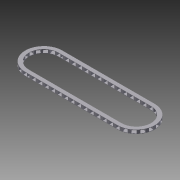
# Autodesk Inventor part: chain
Saved by Autodesk Inventor 2011 (Build 150239000, 239)
## iProperties
Created: 2010-04-19
Part Number: chain
Document SubType Name: Modeling
Designer: lucio
Density: 2.71 g/cm^3
Material: Aluminum-6061
Mass: 13.7583 g
Surface Area: 102.226 cm^2
Volume: 5.07686 cm^3
Author: lucio
Autodesk Inventor part; units mm, degrees
ref_plane "YZ Plane" through (0, 0, 0) normal (1, 0, 0) x (0, 1, 0)
ref_plane "XZ Plane" through (0, 0, 0) normal (0, 1, 0) x (-1, 0, 0)
ref_plane "XY Plane" through (0, 0, 0) normal (0, 0, 1) x (1, 0, 0)
sketch "Sketch1" plane through (0, 0, 0) normal (0, 0, 1) x (1, 0, 0)
  line L0 (25, 0) -> (150, 0)
  line L1 (175, 25) -> (175, 25)
  line L2 (150, 50) -> (25, 50)
  line L3 (0, 25) -> (0, 25)
  arc A0 (25, 50) -> (0, 25) centre (25, 25) ccw
  arc A1 (175, 25) -> (150, 50) centre (150, 25) ccw
  arc A2 (150, 0) -> (175, 25) centre (150, 25) ccw
  arc A3 (0, 25) -> (25, 0) centre (25, 25) ccw
  line L4 (25, 45) -> (150, 45)
  line L5 (170, 25) -> (170, 25)
  line L6 (150, 5) -> (25, 5)
  line L7 (5, 25) -> (5, 25)
  arc A4 (25, 45) -> (5, 25) centre (25, 25) ccw
  arc A5 (5, 25) -> (25, 5) centre (25, 25) ccw
  arc A6 (150, 5) -> (170, 25) centre (150, 25) ccw
  arc A7 (170, 25) -> (150, 45) centre (150, 25) ccw
  line L8 (22.5, 25) -> (27.5, 25)
  line L9 (27.5, 25) -> (27.5, 50)
  line L10 (27.5, 50) -> (22.5, 50)
  line L11 (22.5, 50) -> (22.5, 25)
  line L12 (22.650768, 24.14495) -> (27.349232, 25.85505)
  line L13 (27.349232, 25.85505) -> (18.798728, 49.347366)
  line L14 (18.798728, 49.347366) -> (14.100265, 47.637265)
  line L15 (14.100265, 47.637265) -> (22.650768, 24.14495)
  line L16 (23.084889, 23.393031) -> (26.915111, 26.606969)
  line L17 (26.915111, 26.606969) -> (10.845421, 45.75808)
  line L18 (10.845421, 45.75808) -> (7.015199, 42.544142)
  line L19 (7.015199, 42.544142) -> (23.084889, 23.393031)
  line L20 (23.75, 22.834936) -> (26.25, 27.165064)
  line L21 (26.25, 27.165064) -> (4.599365, 39.665064)
  line L22 (4.599365, 39.665064) -> (2.099365, 35.334936)
  line L23 (2.099365, 35.334936) -> (23.75, 22.834936)
  line L24 (24.56588, 22.537981) -> (25.43412, 27.462019)
  line L25 (25.43412, 27.462019) -> (0.813927, 31.803224)
  line L26 (0.813927, 31.803224) -> (-0.054314, 26.879185)
  line L27 (-0.054314, 26.879185) -> (24.56588, 22.537981)
  line L28 (25.43412, 22.537981) -> (24.56588, 27.462019)
  line L29 (24.56588, 27.462019) -> (-0.054314, 23.120815)
  line L30 (-0.054314, 23.120815) -> (0.813927, 18.196776)
  line L31 (0.813927, 18.196776) -> (25.43412, 22.537981)
  line L32 (26.25, 22.834936) -> (23.75, 27.165064)
  line L33 (23.75, 27.165064) -> (2.099365, 14.665064)
  line L34 (2.099365, 14.665064) -> (4.599365, 10.334936)
  line L35 (4.599365, 10.334936) -> (26.25, 22.834936)
  line L36 (26.915111, 23.393031) -> (23.084889, 26.606969)
  line L37 (23.084889, 26.606969) -> (7.015199, 7.455858)
  line L38 (7.015199, 7.455858) -> (10.845421, 4.24192)
  line L39 (10.845421, 4.24192) -> (26.915111, 23.393031)
  line L40 (27.349232, 24.14495) -> (22.650768, 25.85505)
  line L41 (22.650768, 25.85505) -> (14.100265, 2.362735)
  line L42 (14.100265, 2.362735) -> (18.798728, 0.652634)
  line L43 (18.798728, 0.652634) -> (27.349232, 24.14495)
  line L44 (27.5, 25) -> (22.5, 25)
  line L45 (22.5, 25) -> (22.5, 0)
  line L46 (22.5, 0) -> (27.5, 0)
  line L47 (27.5, 0) -> (27.5, 25)
  line L48 (147.5, 24.96674) -> (152.5, 24.96674)
  line L49 (152.5, 24.96674) -> (152.5, 51.038636)
  line L50 (152.082241, 51.032629) -> (147.5, 50.96674)
  line L51 (147.5, 50.96674) -> (147.5, 24.96674)
  line L52 (147.639393, 25.823796) -> (152.337856, 24.113695)
  line L53 (152.337856, 24.113695) -> (161.254969, 48.613263)
  line L54 (161.254969, 48.613263) -> (156.531917, 50.255804)
  line L55 (156.531917, 50.255804) -> (147.639393, 25.823796)
  line L56 (148.06351, 26.58149) -> (151.893732, 23.367552)
  line L57 (151.893732, 23.367552) -> (168.652423, 43.339783)
  line L58 (168.652423, 43.339783) -> (164.775988, 46.498646)
  line L59 (164.775988, 46.498646) -> (148.06351, 26.58149)
  line L60 (148.721196, 27.148433) -> (151.221196, 22.818306)
  line L61 (151.221196, 22.818306) -> (173.80012, 35.854254)
  line L62 (173.80012, 35.854254) -> (171.237856, 40.148433)
  line L63 (171.237856, 40.148433) -> (148.721196, 27.148433)
  line L64 (149.533125, 27.456244) -> (150.401366, 22.532205)
  line L65 (150.401366, 22.532205) -> (176.077171, 27.059542)
  line L66 (176.077171, 27.059542) -> (175.138126, 31.971096)
  line L67 (175.138126, 31.971096) -> (149.533125, 27.456244)
  line L68 (150.401366, 27.467795) -> (149.533125, 22.543756)
  line L69 (149.533125, 22.543756) -> (175.20893, 18.016419)
  line L70 (175.20893, 18.016419) -> (176.006367, 22.952942)
  line L71 (176.006367, 22.952942) -> (150.401366, 27.467795)
  line L72 (151.221196, 27.181694) -> (148.721196, 22.851567)
  line L73 (148.721196, 22.851567) -> (171.30012, 9.815619)
  line L74 (171.30012, 9.815619) -> (173.737856, 14.181694)
  line L75 (173.737856, 14.181694) -> (151.221196, 27.181694)
  line L76 (151.893732, 26.632448) -> (148.06351, 23.41851)
  line L77 (148.06351, 23.41851) -> (164.822201, 3.446279)
  line L78 (164.822201, 3.446279) -> (168.60621, 6.715292)
  line L79 (168.60621, 6.715292) -> (151.893732, 26.632448)
  line L80 (152.337856, 25.886305) -> (147.639393, 24.176204)
  line L81 (147.639393, 24.176204) -> (156.556506, -0.323364)
  line L82 (156.556506, -0.323364) -> (161.23038, 1.454297)
  line L83 (161.23038, 1.454297) -> (152.337856, 25.886305)
  line L84 (152.5, 25.03326) -> (147.5, 25.03326)
  line L85 (147.5, 25.03326) -> (147.5, -1.038636)
  line L86 (147.5, -1.038636) -> (152.5, -0.96674)
  line L87 (152.5, -0.96674) -> (152.5, 25.03326)
  line L88 (143.785, 50) -> (138.785, 50)
  line L89 (138.785, 50) -> (138.785, -0.715226)
  line L90 (138.785, -0.715226) -> (143.785, -0.715226)
  line L91 (143.785, -0.715226) -> (143.785, 50)
  line L92 (135.07, 50) -> (130.07, 50)
  line L93 (130.07, 50) -> (130.07, 0)
  line L94 (130.07, 0) -> (135.07, 0)
  line L95 (135.07, 0) -> (135.07, 50)
  line L96 (126.355, 0) -> (121.355, 0)
  line L97 (121.355, 0) -> (121.355, 50)
  line L98 (121.355, 50) -> (126.355, 50)
  line L99 (126.355, 50) -> (126.355, 0)
  line L100 (117.64, 50) -> (112.64, 50)
  line L101 (112.64, 50) -> (112.64, 0)
  line L102 (112.64, 0) -> (117.64, 0)
  line L103 (117.64, 0) -> (117.64, 50)
  line L104 (108.925, 50) -> (103.925, 50)
  line L105 (103.925, 50) -> (103.925, 0)
  line L106 (103.925, 0) -> (108.925, 0)
  line L107 (108.925, 0) -> (108.925, 50)
  line L108 (100.21, 50) -> (95.21, 50)
  line L109 (95.21, 50) -> (95.21, 0)
  line L110 (95.21, 0) -> (100.21, 0)
  line L111 (100.21, 0) -> (100.21, 50)
  line L112 (91.495, 50) -> (86.495, 50)
  line L113 (86.495, 50) -> (86.495, 0)
  line L114 (86.495, 0) -> (91.495, 0)
  line L115 (91.495, 0) -> (91.495, 50)
  line L116 (82.78, 50) -> (77.78, 50)
  line L117 (77.78, 50) -> (77.78, 0)
  line L118 (77.78, 0) -> (82.78, 0)
  line L119 (82.78, 0) -> (82.78, 50)
  line L120 (74.065, 50) -> (69.065, 50)
  line L121 (69.065, 50) -> (69.065, 0)
  line L122 (69.065, 0) -> (74.065, 0)
  line L123 (74.065, 0) -> (74.065, 50)
  line L124 (65.35, 50) -> (60.35, 50)
  line L125 (60.35, 50) -> (60.35, 0)
  line L126 (60.35, 0) -> (65.35, 0)
  line L127 (65.35, 0) -> (65.35, 50)
  line L128 (56.635, 50) -> (51.635, 50)
  line L129 (51.635, 50) -> (51.635, 0)
  line L130 (51.635, 0) -> (56.635, 0)
  line L131 (56.635, 0) -> (56.635, 50)
  line L132 (47.92, 50) -> (42.92, 50)
  line L133 (42.92, 50) -> (42.92, 0)
  line L134 (42.92, 0) -> (47.92, 0)
  line L135 (47.92, 0) -> (47.92, 50)
  line L136 (39.205, 50) -> (34.205, 50)
  line L137 (34.205, 50) -> (34.205, 0)
  line L138 (34.205, 0) -> (39.205, 0)
  line L139 (39.205, 0) -> (39.205, 50)
  line L140 (30.49, 50) -> (27.688199, 50)
  line L141 (27.688199, 50) -> (27.688199, 0)
  line L142 (27.688199, 0) -> (30.49, 0)
  line L143 (30.49, 0) -> (30.49, 50)
  line L144 (152.082241, 51.032629) -> (147.5, 51.032629)
  line L145 (147.5, 51.032629) -> (147.5, 25.03326)
  line L146 (147.5, 25.03326) -> (152.082241, 25.03326)
  line L147 (152.082241, 25.03326) -> (152.082241, 51.032629)
  point P0 (0, 0)
  point P1 (175, 50)
  point P2 (175, 0)
  point P3 (0, 50)
  point P4 (170, 5)
  point P5 (170, 45)
  point P6 (5, 5)
  point P7 (16.449496, 48.492316)
  point P8 (18.159597, 43.793852)
  point P9 (8.93031, 44.151111)
  point P10 (12.144248, 40.320889)
  point P11 (3.349365, 37.5)
  point P12 (7.679492, 35)
  point P13 (0.379806, 29.341204)
  point P14 (5.303845, 28.472964)
  point P15 (0.379806, 20.658796)
  point P16 (5.303845, 21.527036)
  point P17 (3.349365, 12.5)
  point P18 (7.679492, 15)
  point P19 (8.93031, 5.848889)
  point P20 (12.144248, 9.679111)
  point P21 (16.449496, 1.507684)
  point P22 (18.159597, 6.206148)
  point P23 (25, 0)
  point P24 (25, 5)
  point P25 (158.550504, 48.492316)
  point P26 (156.840403, 43.793852)
  point P27 (166.06969, 44.151111)
  point P28 (162.855752, 40.320889)
  point P29 (171.650635, 37.5)
  point P30 (167.320508, 35)
  point P31 (174.620194, 29.341204)
  point P32 (169.696155, 28.472964)
  point P33 (174.620194, 20.658796)
  point P34 (169.696155, 21.527036)
  point P35 (171.650635, 12.5)
  point P36 (167.320508, 15)
  point P37 (166.06969, 5.848889)
  point P38 (162.855752, 9.679111)
  point P39 (158.550504, 1.507684)
  point P40 (156.840403, 6.206148)
  point P41 (150, 5)
  dimension "d0" = 175
  dimension "d1" = 50
  dimension "d2" = 25
  dimension "d3" = 165
  dimension "d4" = 40
  dimension "d6" = 20
  dimension "d11" = 2.5
  dimension "d12" = 5
  dimension "d15" = 180
  dimension "d19" = 2.5
  dimension "d20" = 5
  dimension "d23" = 180
  dimension "d27" = 5
  dimension "d28" = 3.715
  dimension "d29" = 3.715
  dimension "d30" = 3.715
  dimension "d31" = 5
  dimension "d32" = 5
  dimension "d33" = 3.715
  dimension "d34" = 5
  dimension "d35" = 3.715
  dimension "d36" = 5
  dimension "d37" = 3.715
  dimension "d38" = 5
  dimension "d39" = 3.715
  dimension "d40" = 5
  dimension "d41" = 3.715
  dimension "d42" = 5
  dimension "d43" = 3.715
  dimension "d44" = 5
  dimension "d45" = 3.715
  dimension "d46" = 5
  dimension "d47" = 3.715
  dimension "d48" = 5
  dimension "d49" = 3.715
  dimension "d50" = 5
  dimension "d51" = 3.715
  dimension "d52" = 5
  dimension "d53" = 2.8018
  dimension "d54" = 3.715
  dimension "d59" = 26
  dimension "d60" = 26
  constraints: 292 end point, 35 parallel, 18 horizontal, 18 perpendicular, 16 point on circle, 12 coincident, 12 tangent, 10 point on line, 8 centre point, 6 equal radius, 1 vertical, 294 other
  measures "d0" distance of point (0, 50) point (175, 50)
  measures "d1" distance of point (175, 50) point (175, 0)
  measures "d2" radius of A0
  measures "d3" distance of point (170, 5) point (5, 5)
  measures "d4" distance of point (170, 45) point (170, 5)
  measures "d6" radius of A4
  measures "d11" distance from line of A0.centre L11
  measures "d12" distance between parallel lines of L11 L9
  measures "d19" distance from line of L51 A1.centre
  measures "d20" distance between parallel lines of L49 L51
  measures "d27" distance between parallel lines of L91 L89
  measures "d28" distance between parallel lines of L51 L91
  measures "d29" distance between parallel lines of L99 L93
  measures "d30" distance between parallel lines of L95 L89
  measures "d31" distance between parallel lines of L93 L95
  measures "d32" distance between parallel lines of L97 L99
  measures "d33" distance between parallel lines of L103 L97
  measures "d34" distance between parallel lines of L101 L103
  measures "d35" distance between parallel lines of L107 L101
  measures "d36" distance between parallel lines of L105 L107
  measures "d37" distance between parallel lines of L111 L105
  measures "d38" distance between parallel lines of L109 L111
  measures "d39" distance between parallel lines of L109 L115
  measures "d40" distance between parallel lines of L113 L115
  measures "d41" distance between parallel lines of L119 L113
  measures "d42" distance between parallel lines of L117 L119
  measures "d43" distance between parallel lines of L123 L117
  measures "d44" distance between parallel lines of L121 L123
  measures "d45" distance between parallel lines of L127 L121
  measures "d46" distance between parallel lines of L125 L127
  measures "d47" distance between parallel lines of L131 L125
  measures "d48" distance between parallel lines of L129 L131
  measures "d49" distance between parallel lines of L135 L129
  measures "d50" distance between parallel lines of L133 L135
  measures "d51" distance between parallel lines of L133 L139
  measures "d52" distance between parallel lines of L137 L139
  measures "d53" distance between parallel lines of L141 L143
  measures "d54" distance between parallel lines of L143 L137
  measures "d59" distance of L50.end L48.start
  measures "d60" distance from line of A1.centre L50
sketch "Sketch1 outline for Extrusion1" plane through (0, 0, 0) normal (0, 0, 1) x (1, 0, 0)
  line L0 (150, 50) -> (25, 50)
  arc A0 (175, 25) -> (150, 50) centre (150, 25) ccw
  arc A1 (25, 50) -> (0, 25) centre (25, 25) ccw
  arc A2 (150, 0) -> (175, 25) centre (150, 25) ccw
  arc A3 (0, 25) -> (25, 0) centre (25, 25) ccw
  line L1 (25, 0) -> (150, 0)
  line L2 (150, 45) -> (25, 45)
  arc A4 (25, 45) -> (5, 25) centre (25, 25) ccw
  arc A5 (5, 25) -> (25, 5) centre (25, 25) ccw
  line L3 (25, 5) -> (150, 5)
  arc A6 (150, 5) -> (170, 25) centre (150, 25) ccw
  arc A7 (170, 25) -> (150, 45) centre (150, 25) ccw
extrude "Extrusion1" add sketch "Sketch1 outline for Extrusion1" along normal mid plane 5
sketch "Sketch1 outline for Extrusion2" plane through (0, 0, 0) normal (0, 0, 1) x (1, 0, 0)
  line L0 (27.5, 0) -> (27.5, 50)
  line L1 (27.5, 50) -> (22.5, 50)
  line L2 (22.5, 50) -> (22.5, 39.178205)
  line L3 (18.798728, 49.347366) -> (22.5, 39.178205)
  line L4 (14.100265, 47.637265) -> (18.798728, 49.347366)
  line L5 (17.801537, 37.468104) -> (14.100265, 47.637265)
  line L6 (10.845421, 45.75808) -> (17.801537, 37.468104)
  line L7 (7.015199, 42.544142) -> (10.845421, 45.75808)
  line L8 (13.971315, 34.254166) -> (7.015199, 42.544142)
  line L9 (4.599365, 39.665064) -> (13.971315, 34.254166)
  line L10 (2.099365, 35.334936) -> (4.599365, 39.665064)
  line L11 (11.471315, 29.924039) -> (2.099365, 35.334936)
  line L12 (0.813927, 31.803224) -> (11.471315, 29.924039)
  line L13 (-0.054314, 26.879185) -> (0.813927, 31.803224)
  line L14 (10.603074, 25) -> (-0.054314, 26.879185)
  line L15 (-0.054314, 23.120815) -> (10.603074, 25)
  line L16 (0.813927, 18.196776) -> (-0.054314, 23.120815)
  line L17 (11.471315, 20.075961) -> (0.813927, 18.196776)
  line L18 (2.099365, 14.665064) -> (11.471315, 20.075961)
  line L19 (4.599365, 10.334936) -> (2.099365, 14.665064)
  line L20 (13.971315, 15.745834) -> (4.599365, 10.334936)
  line L21 (7.015199, 7.455858) -> (13.971315, 15.745834)
  line L22 (10.845421, 4.24192) -> (7.015199, 7.455858)
  line L23 (17.801537, 12.531896) -> (10.845421, 4.24192)
  line L24 (14.100265, 2.362735) -> (17.801537, 12.531896)
  line L25 (18.798728, 0.652634) -> (14.100265, 2.362735)
  line L26 (22.5, 10.821795) -> (18.798728, 0.652634)
  line L27 (22.5, 0) -> (22.5, 10.821795)
  line L28 (27.5, 0) -> (22.5, 0)
extrude "Extrusion2" cut sketch "Sketch1 outline for Extrusion2" along normal mid plane 4
sketch "Sketch1 outline for Extrusion3" plane through (0, 0, 0) normal (0, 0, 1) x (1, 0, 0)
  line L0 (152.082241, 51.032629) -> (147.5, 51.032629)
  line L1 (147.5, 51.032629) -> (147.5, -1.038636)
  line L2 (152.5, -0.96674) -> (147.5, -1.038636)
  line L3 (152.5, 10.821795) -> (152.5, -0.96674)
  line L4 (156.556506, -0.323364) -> (152.5, 10.821795)
  line L5 (161.23038, 1.454297) -> (156.556506, -0.323364)
  line L6 (157.198463, 12.531896) -> (161.23038, 1.454297)
  line L7 (164.822201, 3.446279) -> (157.198463, 12.531896)
  line L8 (168.60621, 6.715292) -> (164.822201, 3.446279)
  line L9 (161.028685, 15.745834) -> (168.60621, 6.715292)
  line L10 (171.30012, 9.815619) -> (161.028685, 15.745834)
  line L11 (173.737856, 14.181694) -> (171.30012, 9.815619)
  line L12 (163.528685, 20.075961) -> (173.737856, 14.181694)
  line L13 (175.20893, 18.016419) -> (163.528685, 20.075961)
  line L14 (176.006367, 22.952942) -> (175.20893, 18.016419)
  line L15 (164.396926, 25) -> (176.006367, 22.952942)
  line L16 (176.077171, 27.059542) -> (164.396926, 25)
  line L17 (175.138126, 31.971096) -> (176.077171, 27.059542)
  line L18 (163.528685, 29.924039) -> (175.138126, 31.971096)
  line L19 (173.80012, 35.854254) -> (163.528685, 29.924039)
  line L20 (171.237856, 40.148433) -> (173.80012, 35.854254)
  line L21 (161.028685, 34.254166) -> (171.237856, 40.148433)
  line L22 (168.652423, 43.339783) -> (161.028685, 34.254166)
  line L23 (164.775988, 46.498646) -> (168.652423, 43.339783)
  line L24 (157.198463, 37.468104) -> (164.775988, 46.498646)
  line L25 (161.254969, 48.613263) -> (157.198463, 37.468104)
  line L26 (156.531917, 50.255804) -> (161.254969, 48.613263)
  line L27 (152.082241, 38.03042) -> (156.531917, 50.255804)
  line L28 (152.082241, 38.03042) -> (152.082241, 51.032629)
extrude "Extrusion3" cut sketch "Sketch1 outline for Extrusion3" along normal mid plane 4
sketch "Sketch1 outline for Extrusion4" plane through (0, 0, 0) normal (0, 0, 1) x (1, 0, 0)
  line L0 (135.07, 50) -> (130.07, 50)
  line L1 (130.07, 50) -> (130.07, 45)
  line L2 (126.355, 45) -> (130.07, 45)
  line L3 (126.355, 45) -> (126.355, 50)
  line L4 (126.355, 50) -> (121.355, 50)
  line L5 (121.355, 50) -> (121.355, 45)
  line L6 (117.64, 45) -> (121.355, 45)
  line L7 (117.64, 45) -> (117.64, 50)
  line L8 (117.64, 50) -> (112.64, 50)
  line L9 (112.64, 50) -> (112.64, 45)
  line L10 (108.925, 45) -> (112.64, 45)
  line L11 (108.925, 45) -> (108.925, 50)
  line L12 (108.925, 50) -> (103.925, 50)
  line L13 (103.925, 50) -> (103.925, 45)
  line L14 (100.21, 45) -> (103.925, 45)
  line L15 (100.21, 45) -> (100.21, 50)
  line L16 (100.21, 50) -> (95.21, 50)
  line L17 (95.21, 50) -> (95.21, 45)
  line L18 (91.495, 45) -> (95.21, 45)
  line L19 (91.495, 45) -> (91.495, 50)
  line L20 (91.495, 50) -> (86.495, 50)
  line L21 (86.495, 50) -> (86.495, 45)
  line L22 (82.78, 45) -> (86.495, 45)
  line L23 (82.78, 45) -> (82.78, 50)
  line L24 (82.78, 50) -> (77.78, 50)
  line L25 (77.78, 50) -> (77.78, 45)
  line L26 (74.065, 45) -> (77.78, 45)
  line L27 (74.065, 45) -> (74.065, 50)
  line L28 (74.065, 50) -> (69.065, 50)
  line L29 (69.065, 50) -> (69.065, 45)
  line L30 (65.35, 45) -> (69.065, 45)
  line L31 (65.35, 45) -> (65.35, 50)
  line L32 (65.35, 50) -> (60.35, 50)
  line L33 (60.35, 50) -> (60.35, 45)
  line L34 (56.635, 45) -> (60.35, 45)
  line L35 (56.635, 45) -> (56.635, 50)
  line L36 (56.635, 50) -> (51.635, 50)
  line L37 (51.635, 50) -> (51.635, 45)
  line L38 (47.92, 45) -> (51.635, 45)
  line L39 (47.92, 45) -> (47.92, 50)
  line L40 (47.92, 50) -> (42.92, 50)
  line L41 (42.92, 50) -> (42.92, 45)
  line L42 (39.205, 45) -> (42.92, 45)
  line L43 (39.205, 45) -> (39.205, 50)
  line L44 (39.205, 50) -> (34.205, 50)
  line L45 (34.205, 50) -> (34.205, 45)
  line L46 (30.49, 45) -> (34.205, 45)
  line L47 (30.49, 45) -> (30.49, 50)
  line L48 (30.49, 50) -> (27.688199, 50)
  line L49 (27.688199, 50) -> (27.688199, 45)
  line L50 (25, 45) -> (27.688199, 45)
  arc A0 (25, 45) -> (25, 5) centre (25, 25) ccw
  line L51 (27.688199, 5) -> (25, 5)
  line L52 (27.688199, 5) -> (27.688199, 0)
  line L53 (27.688199, 0) -> (30.49, 0)
  line L54 (30.49, 0) -> (30.49, 5)
  line L55 (34.205, 5) -> (30.49, 5)
  line L56 (34.205, 5) -> (34.205, 0)
  line L57 (34.205, 0) -> (39.205, 0)
  line L58 (39.205, 0) -> (39.205, 5)
  line L59 (42.92, 5) -> (39.205, 5)
  line L60 (42.92, 5) -> (42.92, 0)
  line L61 (42.92, 0) -> (47.92, 0)
  line L62 (47.92, 0) -> (47.92, 5)
  line L63 (51.635, 5) -> (47.92, 5)
  line L64 (51.635, 5) -> (51.635, 0)
  line L65 (51.635, 0) -> (56.635, 0)
  line L66 (56.635, 0) -> (56.635, 5)
  line L67 (60.35, 5) -> (56.635, 5)
  line L68 (60.35, 5) -> (60.35, 0)
  line L69 (60.35, 0) -> (65.35, 0)
  line L70 (65.35, 0) -> (65.35, 5)
  line L71 (69.065, 5) -> (65.35, 5)
  line L72 (69.065, 5) -> (69.065, 0)
  line L73 (69.065, 0) -> (74.065, 0)
  line L74 (74.065, 0) -> (74.065, 5)
  line L75 (77.78, 5) -> (74.065, 5)
  line L76 (77.78, 5) -> (77.78, 0)
  line L77 (77.78, 0) -> (82.78, 0)
  line L78 (82.78, 0) -> (82.78, 5)
  line L79 (86.495, 5) -> (82.78, 5)
  line L80 (86.495, 5) -> (86.495, 0)
  line L81 (86.495, 0) -> (91.495, 0)
  line L82 (91.495, 0) -> (91.495, 5)
  line L83 (95.21, 5) -> (91.495, 5)
  line L84 (95.21, 5) -> (95.21, 0)
  line L85 (95.21, 0) -> (100.21, 0)
  line L86 (100.21, 0) -> (100.21, 5)
  line L87 (103.925, 5) -> (100.21, 5)
  line L88 (103.925, 5) -> (103.925, 0)
  line L89 (103.925, 0) -> (108.925, 0)
  line L90 (108.925, 0) -> (108.925, 5)
  line L91 (112.64, 5) -> (108.925, 5)
  line L92 (112.64, 5) -> (112.64, 0)
  line L93 (112.64, 0) -> (117.64, 0)
  line L94 (117.64, 0) -> (117.64, 5)
  line L95 (121.355, 5) -> (117.64, 5)
  line L96 (121.355, 5) -> (121.355, 0)
  line L97 (121.355, 0) -> (126.355, 0)
  line L98 (126.355, 0) -> (126.355, 5)
  line L99 (130.07, 5) -> (126.355, 5)
  line L100 (130.07, 5) -> (130.07, 0)
  line L101 (130.07, 0) -> (135.07, 0)
  line L102 (135.07, 0) -> (135.07, 5)
  line L103 (138.785, 5) -> (135.07, 5)
  line L104 (138.785, 5) -> (138.785, -0.715226)
  line L105 (138.785, -0.715226) -> (143.785, -0.715226)
  line L106 (143.785, -0.715226) -> (143.785, 5)
  line L107 (150, 5) -> (143.785, 5)
  arc A1 (150, 5) -> (150, 45) centre (150, 25) ccw
  line L108 (143.785, 45) -> (150, 45)
  line L109 (143.785, 45) -> (143.785, 50)
  line L110 (143.785, 50) -> (138.785, 50)
  line L111 (138.785, 50) -> (138.785, 45)
  line L112 (135.07, 45) -> (138.785, 45)
  line L113 (135.07, 45) -> (135.07, 50)
extrude "Extrusion4" cut sketch "Sketch1 outline for Extrusion4" along normal mid plane 4
equation "\"d29\" = d28"
equation "\"d30\" = d28"
equation "\"d31\" = d27"
equation "\"d32\" = d20"
equation "\"d33\" = d28"
equation "\"d34\" = d27"
equation "\"d35\" = d28"
equation "\"d36\" = d20"
equation "\"d37\" = d28"
equation "\"d38\" = d20"
equation "\"d39\" = d28"
equation "\"d40\" = d20"
equation "\"d41\" = d28"
equation "\"d42\" = d20"
equation "\"d43\" = d28"
equation "\"d44\" = d20"
equation "\"d45\" = d28"
equation "\"d46\" = d20"
equation "\"d47\" = d28"
equation "\"d48\" = d20"
equation "\"d49\" = d28"
equation "\"d50\" = d20"
equation "\"d51\" = d28"
equation "\"d52\" = d20"
equation "\"d54\" = d28"
body "Solid1"
